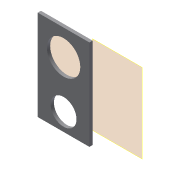
# Autodesk Inventor part: 200_Gearbox_conterplate
Saved by Autodesk Inventor 2019 (Build 230136000, 136)
## iProperties
Created: 2019-07-08
Part Number: 200_Gearbox_conterplate
Material: Generic
Document SubType Name: Modeling
Designer: diederichbenedict
Density: 1 g/cm^3
Appearance: Default
Author: diederichbenedict
Autodesk Inventor part; units mm, degrees
ref_plane "YZ Plane" through (0, 0, 0) normal (1, 0, 0) x (0, 1, 0)
ref_plane "XZ Plane" through (0, 0, 0) normal (0, 1, 0) x (-1, 0, 0)
ref_plane "XY Plane" through (0, 0, 0) normal (0, 0, 1) x (1, 0, 0)
ref_plane "Work Plane1" through (0, 0, 0) normal (0, 0, 1) x (1, 0, 0)
ref_plane "Work Plane2" through (-27.9392, 13.2515, 3.3744) normal (0, 0, 1) x (0.9999936, 0.0035868, 0)
sketch "Sketch4" plane through (-27.9392, 13.2515, 3.3744) normal (0, 0, 1) x (0.9999936, 0.0035868, 0)
  circle A0 centre (0.0013, -0.0001) radius 12.5 construction
  line L0 (17.0013, 16.9999) -> (-16.9987, 16.9999) construction
  line L1 (-16.9987, 16.9999) -> (-16.9987, -40.0001) construction
  line L2 (-16.9987, -40.0001) -> (17.0013, -40.0001) construction
  line L3 (17.0013, -40.0001) -> (17.0013, 16.9999) construction
  line L4 (17.0013, 16.9999) -> (-16.9987, 16.9999)
  line L5 (-16.9987, 16.9999) -> (-16.9987, -40.0001)
  line L6 (-16.9987, -40.0001) -> (17.0013, -40.0001)
  line L7 (17.0013, -40.0001) -> (17.0013, 16.9999)
  circle A1 centre (0.0013, -0.0001) radius 10.3271
  circle A2 centre (-0.1451, -29.1987) radius 12.8 construction
  circle A3 centre (-0.1034, -29.1986) radius 8.1726 construction
  circle A4 centre (-0.1034, -29.1986) radius 8
  point P0 (27.8915, -13.3516)
  dimension "d13" = 17
  dimension "d14" = 17
  dimension "d15" = 17
  dimension "d16" = 40
  dimension "d17" = 16
  constraints: 16 end point, 4 parallel, 3 centre point, 2 coincident, 2 horizontal, 2 perpendicular
  measures "d13" distance from line of A0.centre L3
  measures "d14" distance from line of L1 A0.centre
  measures "d15" distance from line of A0.centre L0
  measures "d16" distance from line of A0.centre L2
  measures "d17" diameter of A4
extrude "Extrusion4" add sketch "Sketch4" along normal blind 2
sketch "Sketch5" plane through (-27.9392, 13.2515, 3.3744) normal (0, 0, -1) x (-0.9999936, -0.0035868, 0)
  line L0 (15.2891, -0.4637) -> (15.1772, -1.9039) construction
  circle A0 centre (-0.0013, -0.0001) radius 12.5 construction
  line L1 (15.4007, -29.1278) -> (15.3392, -30.5711) construction
  circle A1 centre (-0.0013, -0.0001) radius 10.3271 construction
  circle A2 centre (0.1034, -29.1986) radius 8 construction
  line L2 (-17.0013, 16.9999) -> (16.9987, 16.9999) construction
  line L3 (-17.0013, -40.0001) -> (-17.0013, 16.9999) construction
  line L4 (16.9987, -40.0001) -> (-17.0013, -40.0001) construction
  line L5 (16.9987, 16.9999) -> (16.9987, -40.0001) construction
  line L6 (16.9987, 16.9999) -> (-17.0013, 16.9999)
  line L7 (-17.0013, 16.9999) -> (-17.0013, -40.0001)
  line L8 (-17.0013, -40.0001) -> (16.9987, -40.0001)
  line L9 (16.9987, -40.0001) -> (16.9987, 16.9999)
  circle A3 centre (-0.0013, -0.0001) radius 15.2975 construction
  arc A4 (5.9476, -14.6347) -> (-5.8452, -14.677) centre (-0.0013, -0.0001) ccw
  arc A5 (-5.1414, -14.4082) -> (5.2419, -14.371) centre (0.1034, -29.1986) ccw
  line L10 (16.9987, -40.0001) -> (-17.0013, -40.0001) projected
  point P0 (-27.8915, -13.3516)
  point P1 (10.9564, -8.3909)
  point P2 (11.4871, -40.0001)
  point P3 (-11.2803, -40.0001)
  dimension "d20" = 0.5
  constraints: 11 point on circle, 8 end point, 3 centre point, 2 coincident, 2 parallel, 2 point on line, 1 horizontal, 1 perpendicular, 1 other
  measures "d20" radial gap between concentric circles of A3 A4
extrude "Extrusion5" add sketch "Sketch5" along normal blind 7 contours L9 L8 A5 A4 L7 L6
sketch "Sketch6" plane through (-27.9392, 13.2515, -3.6256) normal (0, 0, -1) x (-0.9999936, -0.0035868, 0)
  line L0 (16.9987, 16.9999) -> (-17.0013, 16.9999) projected
  line L1 (-17.0013, 16.9999) -> (-17.0013, -40.0001) projected
  line L2 (-17.0013, -40.0001) -> (-11.2803, -40.0001) projected
  arc A0 (-5.8452, -14.677) -> (-11.2803, -40.0001) centre (0.1034, -29.1986) ccw projected
  arc A1 (5.9476, -14.6347) -> (-5.8452, -14.677) centre (-0.0013, -0.0001) ccw projected
  arc A2 (11.4871, -40.0001) -> (5.9476, -14.6347) centre (0.1034, -29.1986) ccw projected
  line L3 (11.4871, -40.0001) -> (16.9987, -40.0001) projected
  line L4 (16.9987, -40.0001) -> (16.9987, 16.9999) projected
  point P0 (-27.8915, -13.3516)
  point P1 (14.2429, 13.4801)
  point P2 (14.2429, -14.6347)
  point P3 (-13.5758, -14.6347)
  point P4 (-13.5758, 13.4801)
hole "Hole1" at (-42.2304, 26.6804, -3.6256) at (-42.1296, -1.4342, -3.6256) at (-14.311, -1.3344, -3.6256) at (-14.4119, 26.7802, -3.6256) direction (0, 0, 1) diameter 2.9 depth 24 tip angle 118
body "Solid2"
